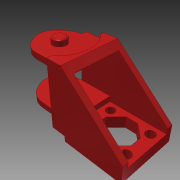
# Autodesk Inventor part: x_axis_cable_mount_b
Saved by Autodesk Inventor 2014 (Build 180170000, 170)
## iProperties
Created: 2013-12-04
Part Number: x_axis_cable_mount_b
Material: ABS Plastic
Document SubType Name: Modeling
Designer: buben
Density: 1.06 g/cm^3
Appearance: Light Red
Author: buben
Autodesk Inventor part; units mm, degrees
ref_plane "YZ Plane" through (0, 0, 0) normal (1, 0, 0) x (0, 1, 0)
sketch "Sketch1" plane through (0, 0, 0) normal (0, 0, 1) x (1, 0, 0)
  circle A0 centre (0, 0) radius 2.5
  circle A1 centre (20, 0) radius 2.5
  line L0 (7, 10) -> (20, 10)
  line L1 (7, -10) -> (20, -10)
  arc A2 (20, -10) -> (20, 10) centre (20, 0) ccw
  line L2 (7, 10) -> (7, 8)
  line L3 (7, -10) -> (7, -8)
  line L4 (7, 8) -> (0, 8)
  line L5 (7, -8) -> (0, -8)
  arc A3 (0, 8) -> (0, -8) centre (0, 0) ccw
  dimension "d0" = 5
  dimension "d1" = 20
  dimension "d2" = 10
  dimension "d3" = 2
  dimension "d4" = 13
  constraints: 12 end point, 4 centre point, 4 point on circle, 4 tangent, 3 parallel, 2 collinear, 2 concentric, 1 coincident, 1 equal radius, 1 horizontal, 1 horizontal alignment, 1 perpendicular
  measures "d0" diameter of A0
  measures "d1" distance of A1.centre point (0, 0)
  measures "d2" radius of A2
  measures "d3" distance of L0.start L2.end
  measures "d4" distance from line of L2 A1.centre
extrude "Extrusion1" add sketch "Sketch1" along normal blind 4
sketch "Sketch2" plane through (0, 0, 4) normal (0, 0, 1) x (1, 0, 0)
  circle A0 centre (0, 0) radius 2.5 projected
  line L0 (7, 8) -> (0, 8) projected
  arc A1 (0, 8) -> (0, -8) centre (0, 0) ccw projected
  line L1 (0, -8) -> (7, -8) projected
  line L2 (7, -10) -> (20, -10) projected
  line L3 (7, 8) -> (7, -8)
  line L4 (7, -8) -> (0, -8)
  line L5 (7, 8) -> (0, 8)
  arc A2 (0, 8) -> (0, -8) centre (0, 0) ccw
  constraints: 6 end point, 4 tangent, 2 collinear, 2 point on circle, 1 centre point, 1 perpendicular
extrude "Extrusion2" cut sketch "Sketch2" against normal blind 2
sketch "Sketch3" plane through (0, 0, 0) normal (0, 0, -1) x (-1, 0, 0)
  circle A0 centre (-20, 0) radius 2.5 projected
  circle A1 centre (0, 0) radius 2.5 projected
  line L0 (-7, 10) -> (-20, 10) projected
  arc A2 (-20, 10) -> (-20, -10) centre (-20, 0) ccw projected
  line L1 (-20, -10) -> (-7, -10) projected
  line L2 (-7, 8) -> (-7, 10) projected
  line L3 (-19, 10) -> (-19, 8)
  line L4 (-19, 8) -> (-11, 8)
  line L5 (-11, 8) -> (-11, -8)
  line L6 (-11, -8) -> (-19, -8)
  line L7 (-19, -8) -> (-19, -10)
  point P0 (-7, -8)
  dimension "d9" = 1
  dimension "d10" = 11
  constraints: 10 end point, 3 parallel, 2 horizontal alignment, 2 perpendicular, 2 point on line, 1 collinear
  measures "d9" distance from line of L3 A0.centre
  measures "d10" distance from line of A1.centre L5
extrude "Extrusion3" cut sketch "Sketch3" against normal blind 2 contours L3 L4 L5 L6 L7 L1 A2 L0
sketch "Sketch4" plane through (0, 0, 4) normal (0, 0, 1) x (1, 0, 0)
  line L0 (7, 10) -> (7, -10)
  circle A0 centre (0, 0) radius 2.5
  arc A1 (7, -8.485281) -> (7, 8.485281) centre (0, 0) ccw
  dimension "d15" = 11
  constraints: 2 point on circle, 2 point on line, 1 centre point, 1 coincident
  measures "d15" radius of A1
extrude "Extrusion4" cut sketch "Sketch4" against normal blind 2 contours A1 L0
sketch "Sketch5" plane through (0, 0, 0) normal (0, 0, -1) x (-1, 0, 0)
  line L0 (0, 8) -> (-7, 8) projected
  line L1 (-7, 10) -> (0, 10)
  line L2 (0, 10) -> (0, 8)
  line L3 (0, 8) -> (-7, 8)
  line L4 (-7, 8) -> (-7, 10)
  arc A0 (0, -8) -> (0, 8) centre (0, 0) ccw projected
  constraints: 8 end point, 2 parallel, 1 horizontal, 1 perpendicular, 1 point on line, 1 vertical alignment
extrude "Extrusion5" add sketch "Sketch5" against normal blind 2
sketch "Sketch6" plane through (0, 0, 0) normal (0, 0, -1) x (-1, 0, 0)
  line L0 (0, 10) -> (-19, 10) projected
  line L1 (-19, 8) -> (-20, 8)
  line L2 (-20, 8) -> (-20, 10)
  line L3 (-20, 10) -> (-19, 10)
  line L4 (-19, 10) -> (-19, 8)
  circle A0 centre (-20, 0) radius 2.5 projected
  constraints: 8 end point, 2 parallel, 1 collinear, 1 horizontal, 1 perpendicular, 1 vertical alignment
extrude "Extrusion6" add sketch "Sketch6" against normal blind 2 contours L1 L2 L3 L4
sketch "Sketch7" plane through (0, 0, 0) normal (0, 0, -1) x (-1, 0, 0)
  line L0 (-19, -8) -> (-19, -10)
  line L1 (-11, -8) -> (-19, -8)
  line L2 (-17.400642, -8) -> (-19, -9.162001)
  line L3 (-17.400642, -8) -> (-26.805206, 4.944272) construction
  line L4 (-26.805206, 4.944272) -> (-28.404564, 3.782271) construction
  line L5 (-28.404564, 3.782271) -> (-19, -9.162001) construction
  circle A0 centre (-20, 0) radius 2.5
  line L6 (-17.400642, -8) -> (-19, -8)
  line L7 (-19, -8) -> (-19, -9.162001)
  dimension "d21" = 16
  dimension "d22" = 8
  dimension "d23" = 36
  constraints: 12 end point, 3 perpendicular, 2 point on line, 1 collinear, 1 parallel
  measures "d21" distance of L2.start L3.end
  measures "d22" distance from line of A0.centre L4
  measures "d23" angle of L2 L1
extrude "Extrusion7" cut sketch "Sketch7" against normal blind 2 contours L1 L2 L0
sketch "Sketch9" plane through (0, 0, 2) normal (0, 0, 1) x (1, 0, 0)
  circle A0 centre (0, 0) radius 2.5
  arc A1 (11, 0) -> (7, 8.485281) centre (0, 0) ccw
  circle A2 centre (0, 0) radius 2.5
  constraints: 1 centre point, 1 coincident, 1 concentric
extrude "Extrusion8" add sketch "Sketch9" along normal mid plane 4
fillet "Fillet1" radius 0.5 1 edges at (-2.5, 0, 4)
sketch "Sketch10" plane through (0, 0, 0) normal (0, 0, -1) x (-1, 0, 0)
  arc A0 (0, -8) -> (0, 8) centre (0, 0) ccw
  line L0 (0, 10) -> (-20, 10)
  line L1 (4.702282, 6.472136) -> (11.174418, 1.769854)
  line L2 (11.174418, 1.769854) -> (6.472136, -4.702282)
  dimension "d30" = 144
  constraints: 4 end point, 2 point on circle, 2 tangent, 1 perpendicular
  measures "d30" angle of L1 L0
extrude "Extrusion9" add sketch "Sketch10" against normal blind 2
fillet "Fillet2" radius 6 1 edges at (-11.1744, 1.7699, 1)
ref_plane "Work Plane1" through (11, 0, 4) normal (1, 0, 0) x (0, 1, 0)
split "Split1" plane through (11, 0, 4) removes the side toward (1, 0, 0)
sketch "Sketch11" plane through (11, -10, 0) normal (1, 0, 0) x (0, 0, -1)
  line L0 (0, 20) -> (0, 0) projected
  line L1 (-4, 20) -> (0, 20) projected
  line L2 (-4, 10) -> (-4, 20) projected
  line L3 (-4, 0) -> (-4, 10) projected
  line L4 (0, 0) -> (-4, 0) projected
  point P0 (0, 10)
extrude "Extrusion10" add sketch "Sketch11" along normal blind 1
ref_plane "Work Plane2" through (0, 0, -7) normal (0, 0, -1) x (-1, 0, 0)
mirror "Mirror1" about plane through (0, 0, -7) normal (0, 0, -1)
sketch "Sketch12" plane through (0, 0, 0) normal (0, 0, -1) x (-1, 0, 0)
  line L0 (-12, -10) -> (-7, -10)
  line L1 (-7, -10) -> (-7, -8)
  arc A0 (4.702282, 6.472136) -> (0, 8) centre (0, 0) ccw
  line L2 (0, 8) -> (0, 10)
  line L3 (0, 10) -> (-12, 10)
  line L4 (-12, -10) -> (-12, 10)
  line L5 (0, 8) -> (-12, 8)
  line L6 (-7, -8) -> (-12, -8)
  constraints: 4 end point, 2 perpendicular, 2 point on line, 1 tangent
extrude "Extrusion11" add sketch "Sketch12" along normal blind 14
sketch "Sketch13" plane through (12, -10, 0) normal (1, 0, 0) x (0, 0, -1)
  line L0 (0, 18) -> (14, 18) projected
  line L1 (0, 2) -> (14, 2) projected
  line L2 (-4, 0) -> (18, 0) projected
  line L3 (18, 20) -> (18, 0) projected
  line L4 (-4, 20) -> (18, 20) projected
  line L5 (-4, 20) -> (-4, 0) projected
  line L6 (-2, 18) -> (16, 18)
  line L7 (16, 18) -> (16, 2)
  line L8 (16, 2) -> (-2, 2)
  line L9 (-2, 2) -> (-2, 18)
  point P0 (0, 10)
  dimension "d39" = 2
  dimension "d40" = 2
  constraints: 8 end point, 2 collinear, 2 parallel, 1 horizontal, 1 perpendicular
  measures "d39" distance between parallel lines of L5 L9
  measures "d40" distance between parallel lines of L3 L7
extrude "Extrusion12" add sketch "Sketch13" along normal blind 20
sketch "Sketch14" plane through (7, 10, 4) normal (0, 1, 0) x (1, 0, 0)
  line L0 (25, 0) -> (0, 0) projected
  line L1 (25, 22) -> (25, 0) projected
  line L2 (5, 0) -> (25, 18)
  point P0 (-7, 4)
  dimension "d43" = 4
  dimension "d44" = 20
  constraints: 2 end point, 2 point on line
  measures "d43" distance of L1.start L2.end
  measures "d44" distance of L0.start L2.start
extrude "Extrusion13" cut sketch "Sketch14" against normal blind 20
sketch "Sketch15" plane through (12, -8, -16) normal (0, 0, 1) x (1, 0, 0)
  line L0 (0, 0) -> (0, 16) projected
  line L1 (0, 0) -> (20, 0) projected
  line L2 (20, 16) -> (20, 0) projected
  line L3 (0, 16) -> (20, 16) projected
  line L4 (3, 13) -> (17, 13) construction
  line L5 (17, 13) -> (17, 3) construction
  line L6 (17, 3) -> (3, 3) construction
  line L7 (3, 3) -> (3, 13) construction
  line L8 (8, 14) -> (12, 14)
  line L9 (16, 10) -> (16, 6)
  line L10 (12, 2) -> (8, 2)
  line L11 (4, 6) -> (4, 10)
  line L12 (8, 14) -> (4, 10)
  line L13 (8, 2) -> (4, 6)
  line L14 (12, 2) -> (16, 6)
  line L15 (16, 10) -> (12, 14)
  circle A0 centre (3, 13) radius 1.6
  circle A1 centre (3, 3) radius 1.6
  circle A2 centre (17, 3) radius 1.6
  circle A3 centre (17, 13) radius 1.6
  point P0 (-12, 8)
  point P1 (16, 14)
  point P2 (4, 8)
  point P3 (3, 8)
  dimension "d55" = 3.2
  dimension "d56" = 3
  dimension "d57" = 3
  dimension "d58" = 3
  dimension "d59" = 3
  dimension "d60" = 1
  dimension "d63" = 1
  dimension "d66" = 45
  dimension "d67" = 4
  dimension "d68" = 4
  dimension "d69" = 4
  constraints: 24 end point, 7 perpendicular, 4 centre point, 4 coincident, 4 parallel, 3 equal radius, 2 horizontal, 2 midpoint, 2 point on line, 1 horizontal alignment
  measures "d55" diameter of A0
  measures "d56" distance between parallel lines of L2 L5
  measures "d57" distance between parallel lines of L3 L4
  measures "d58" distance between parallel lines of L1 L6
  measures "d59" distance between parallel lines of L0 L7
  measures "d60" distance between parallel lines of L7 L11
  measures "d63" distance between parallel lines of L5 L9
  measures "d66" angle of L10 L13
  measures "d67" distance of L11.start L11.end
  measures "d68" distance of L8.start L8.end
  measures "d69" distance of L10.start L10.end
extrude "Extrusion14" cut sketch "Sketch15" against normal through all contours L8 L15 L9 L14 L10 L13 L11 L12 | A0 | A1 | A2 | A3
sketch "Sketch16" plane through (0, 0, -18) normal (0, 0, -1) x (-1, 0, 0)
  circle A0 centre (-29, 5) radius 1.6 projected
  circle A1 centre (-15, -5) radius 1.6 projected
  circle A2 centre (-15, 5) radius 1.6 projected
  circle A3 centre (-29, -5) radius 1.6 projected
  line L0 (-16, 2) -> (-16, -2) projected
  line L1 (-16, -2) -> (-20, -6) projected
  line L2 (-20, -6) -> (-24, -6) projected
  line L3 (-24, -6) -> (-28, -2) projected
  line L4 (-28, -2) -> (-28, 2) projected
  line L5 (-28, 2) -> (-24, 6) projected
  line L6 (-24, 6) -> (-20, 6) projected
  line L7 (-20, 6) -> (-16, 2) projected
  line L8 (-7, -10) -> (-32, -10) projected
  line L9 (-32, 10) -> (-12, 10)
  line L10 (-12, 10) -> (-12, -10)
  line L11 (-12, -10) -> (-32, -10)
  line L12 (-32, -10) -> (-32, 10)
  dimension "d70" = 20
  constraints: 8 end point, 2 parallel, 1 horizontal, 1 perpendicular, 1 point on line
  measures "d70" distance between parallel lines of L12 L10
extrude "Extrusion15" add sketch "Sketch16" along normal blind 2
body "Solid1"
